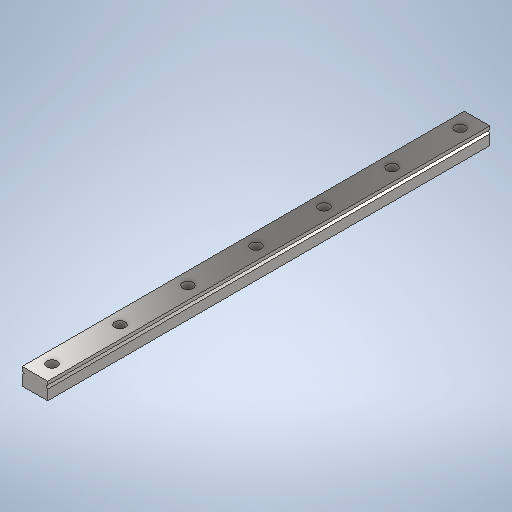
# Autodesk Inventor part: MGN15 Rail Middle
Saved by Autodesk Inventor 2026.2 (Build 302298010, 298A)
## iProperties
Created: 2026-04-28
Part Number: MGN15 Rail Middle
Material: Stainless Steel, 440C
Document SubType Name: Modeling
Designer: chanh
Density: 7.75 g/cm^3
Appearance: Semi-Polished
Author: chanh
Autodesk Inventor part; units mm, degrees
ref_plane "YZ Plane" through (0, 0, 0) normal (1, 0, 0) x (0, 1, 0)
ref_plane "XZ Plane" through (0, 0, 0) normal (0, 1, 0) x (-1, 0, 0)
ref_plane "XY Plane" through (0, 0, 0) normal (0, 0, 1) x (1, 0, 0)
sketch "Sketch1" plane through (0, 0, 0) normal (0, 0, 1) x (1, 0, 0)
  line L0 (-7.5, 5) -> (7.5, 5)
  line L1 (7.5, 5) -> (7.5, -5)
  line L2 (7.5, -5) -> (-7.5, -5)
  line L3 (-7.5, -5) -> (-7.5, 5)
  line L4 (-7.5, 5) -> (7.5, -5) construction
  line L5 (7.5, 5) -> (-7.5, -5) construction
  line L6 (-7.5, 3.0607) -> (-6.4393, 2)
  line L7 (-7.5, 3.0607) -> (-6, 3.0607) construction
  line L8 (-6.4393, 2) -> (-7.5, 0.9393)
  line L9 (0, 5) -> (0, -5) construction
  line L10 (7.5, 3.0607) -> (6.4393, 2)
  line L11 (6.4393, 2) -> (7.5, 0.9393)
  point P0 (0, 0)
  point P1 (7.5, 0.9393)
  point P2 (7.5, 3.0607)
  dimension "d0" = 15
  dimension "d1" = 10
  dimension "d2" = 45
  dimension "d3" = 3
  dimension "d4" = 1.5
  constraints: 24 end point, 4 midpoint, 3 symmetric about line, 2 horizontal, 2 parallel, 2 perpendicular, 2 point on line, 1 equal length
  measures "d0" distance of L1.end L2.end
  measures "d1" distance of L0.end L1.end
  measures "d2" angle of L6 L7
  measures "d3" distance from line of L0 L6.end
  measures "d4" distance of L6.start L6.end
extrude "Extrusion1" add sketch "Sketch1" along normal mid plane 260 contours L0 L1 L10 L11 L2 L3 L8 L6
sketch "Sketch2" plane through (-7.5, 5, 130) normal (0, 1, 0) x (1, 0, 0)
  point P0 (7.5, 130)
  point P1 (7.5, 130)
  constraints: 1 coincident
hole "Hole1" at (0, 5, 0) direction (0, -1, 0) diameter 3.5 end through all counterbore diameter 6 counterbore depth 4.5
pattern_linear "Rectangular Pattern1" count 7 spacing 40 along (0, 0, 1) of "Hole1" first direction both ways yes
sketch "Sketch4" plane through (-7.5, 5, 130) normal (0, 1, 0) x (1, 0, 0)
  circle A0 centre (7.5, 250) radius 3 projected
  circle A1 centre (7.5, 10) radius 3 projected
  point P0 (7.5, 130)
hole "Hole3" at (0, 5, 120) at (0, 5, -120) direction (0, -1, 0) diameter 6 end through all
body "Solid1"
